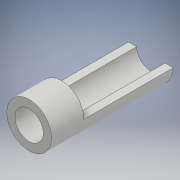
# Autodesk Inventor part: espaciador2
Saved by Autodesk Inventor 2018 (Build 220112000, 112)
## iProperties
Created: 2017-09-07
Part Number: espaciador2
Material: Generic
Document SubType Name: Modeling
Designer: Vidal Villegas
Density: 1 g/cm^3
Appearance: Default
Author: Vidal Villegas
Autodesk Inventor part; units mm, degrees
ref_plane "YZ Plane" through (0, 0, 0) normal (1, 0, 0) x (0, 1, 0)
ref_plane "XZ Plane" through (0, 0, 0) normal (0, 1, 0) x (-1, 0, 0)
ref_plane "XY Plane" through (0, 0, 0) normal (0, 0, 1) x (1, 0, 0)
sketch "Sketch1" plane through (0, 0, 0) normal (0, 1, 0) x (-1, 0, 0)
  circle A0 centre (0, 0) radius 1.75
  circle A1 centre (0, 0) radius 2.75
  dimension "d0" = 3.5
  dimension "d1" = 5.5
  constraints: 2 centre point, 2 coincident
  measures "d0" diameter of A0
  measures "d1" diameter of A1
extrude "Extrusion1" add sketch "Sketch1" along normal blind 4
sketch "Sketch2" plane through (0, 4, 0) normal (0, 1, 0) x (1, 0, 0)
  circle A0 centre (0, 0) radius 1.75 projected
  circle A1 centre (0, 0) radius 2.75 projected
  circle A2 centre (0, 0) radius 2.75
  circle A3 centre (0, 0) radius 1.75
  circle A4 centre (0, 0) radius 2.75 projected
  circle A5 centre (0, 0) radius 1.75 projected
  circle A6 centre (0, 0) radius 2.75 projected
  line L0 (-2.75, 0) -> (0, 0)
  line L1 (0, 0) -> (2.75, 0)
  arc A7 (1.75, 0) -> (-1.75, 0) centre (0, 0) ccw
  arc A8 (2.75, 0) -> (-2.75, 0) centre (0, 0) ccw
  constraints: 8 point on circle, 4 centre point, 4 end point, 3 concentric, 3 point on line, 2 coincident, 1 horizontal
extrude "Extrusion2" add sketch "Sketch2" along normal blind 11 contours A0 L0 A1 L1 picked at (-2.3731, 0.359)
body "Solid1"
